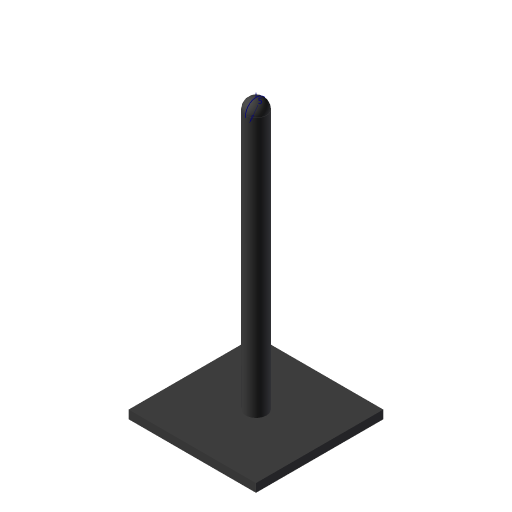
# Autodesk Inventor part: Pivot
Saved by Autodesk Inventor 2023.4 (Build 274418000, 418)
## iProperties
Created: 2024-03-15
Part Number: Pivot
Material: Generic
Document SubType Name: Modeling
Designer: josep
Density: 1 g/cm^3
Appearance: Default
Author: josep
Autodesk Inventor part; units mm, degrees
ref_plane "YZ Plane" through (0, 0, 0) normal (1, 0, 0) x (0, 1, 0)
ref_plane "XZ Plane" through (0, 0, 0) normal (0, 1, 0) x (-1, 0, 0)
ref_plane "XY Plane" through (0, 0, 0) normal (0, 0, 1) x (1, 0, 0)
sketch "Sketch1" plane through (0, 0, 0) normal (0, 1, 0) x (-1, 0, 0)
  line L0 (15, 15) -> (-15, 15)
  line L1 (-15, 15) -> (-15, -15)
  line L2 (-15, -15) -> (15, -15)
  line L3 (15, -15) -> (15, 15)
  point P0 (0, 0)
  point P1 (15, 0)
  point P2 (0, 15)
  dimension "d0" = 30
  dimension "d1" = 30
  dimension "d2" = 0
  dimension "d3" = 0
  constraints: 8 end point, 2 midpoint, 2 parallel, 1 horizontal, 1 perpendicular
  measures "d0" distance of L0.start L0.end
  measures "d1" distance of L2.end L0.start
  measures "d2" vertical distance of point (15, 0) point (0, 0)
  measures "d3" horizontal distance of point (0, 15) point (0, 0)
extrude "Extrusion1" add sketch "Sketch1" along normal blind 2
sketch "Sketch2" plane through (0, 2, 0) normal (0, 1, 0) x (1, 0, 0)
  circle A0 centre (0, 0) radius 2.5
  dimension "d6" = 5
  constraints: 1 centre point, 1 coincident
  measures "d6" diameter of A0
extrude "Extrusion2" add sketch "Sketch2" along normal blind 61.394
sketch "Sketch3" plane through (0, 63.394, 0) normal (0, 1, 0) x (1, 0, 0)
  point P0 (0, 0)
sketch "Sketch4" plane through (0, 0, 0) normal (1, 0, 0) x (0, 1, 0)
  line L0 (63.394, -2.5) -> (63.394, 2.5) projected
  circle A0 centre (63.394, 0) radius 2.5
  line L1 (65.894, 0) -> (63.394, 0)
  line L2 (63.394, 0) -> (63.394, -2.5)
  line L3 (65.894, 0) -> (66.7994, 0)
  point P0 (0, 0)
  dimension "d6" = 5
  dimension "d9" = 5
  constraints: 6 end point, 1 coincident, 1 collinear, 1 horizontal, 1 midpoint, 1 perpendicular, 3 other
revolve "Revolution3" add sketch "Sketch4" angle 360 about axis through (0, 65.894, 0) along (0, -1, 0) picked at (64.2751, -1.4023) contours L0 L1 A0
body "Solid1"
